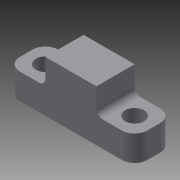
# Autodesk Inventor part: Mirror
Saved by Autodesk Inventor 2015 (Build 190159000, 159)
## iProperties
Created: 2017-12-15
Part Number: Mirror
Material: Generic
Document SubType Name: Modeling
Designer: Administrator
Density: 1 g/cm^3
Appearance: Default
Author: Administrator
Autodesk Inventor part; units mm, degrees
ref_plane "YZ Plane" through (0, 0, 0) normal (1, 0, 0) x (0, 1, 0)
ref_plane "XZ Plane" through (0, 0, 0) normal (0, 1, 0) x (-1, 0, 0)
ref_plane "XY Plane" through (0, 0, 0) normal (0, 0, 1) x (1, 0, 0)
sketch "Sketch1" plane through (0, 0, 0) normal (0, 0, 1) x (1, 0, 0)
  line L0 (0, 0) -> (0, 12.7)
  line L1 (0, 12.7) -> (19.05, 12.7)
  line L2 (19.05, 12.7) -> (19.05, 25.4)
  line L3 (19.05, 25.4) -> (31.75, 25.4)
  line L4 (31.75, 25.4) -> (31.75, 0)
  line L5 (31.75, 0) -> (0, 0)
  dimension "d0" = 12.7
  dimension "d1" = 31.75
  dimension "d2" = 19.05
  dimension "d3" = 12.7
  constraints: 12 end point, 4 perpendicular, 1 vertical
  measures "d0" distance of L0.start L0.end
  measures "d1" distance of L4.end L0.start
  measures "d2" distance of L0.end L1.end
  measures "d3" distance of L1.end L2.end
extrude "Extrusion1" add sketch "Sketch1" along normal blind 19.05
sketch "Sketch2" plane through (0, 12.7, 0) normal (0, 1, 0) x (1, 0, 0)
  line L0 (0, 0) -> (0, -19.05) projected
  line L1 (0, 0) -> (19.05, 0) projected
  point P0 (9.525, -9.525)
  dimension "d6" = 9.525
  dimension "d7" = 9.525
  measures "d6" distance from line of L0 point (9.525, -9.525)
  measures "d7" distance from line of L1 point (9.525, -9.525)
hole "Hole1" at (9.525, 12.7, 9.525) direction (0, -1, 0) diameter 9.525 end through all
fillet "Fillet1" radius 6.35 1 edges at (0, 6.35, 19.05)
fillet "Fillet2" radius 6.35 1 edges at (0, 6.35, 0)
mirror "Mirror1" about plane through (31.75, 0, 0) normal (1, 0, 0) of "Extrusion1", "Hole1", "Fillet1", "Fillet2"
fillet "Fillet3" radius 3.175 1 edges at (44.45, 12.7, 9.525)
fillet "Fillet4" radius 3.175 1 edges at (19.05, 12.7, 9.525)
body "Solid1"
